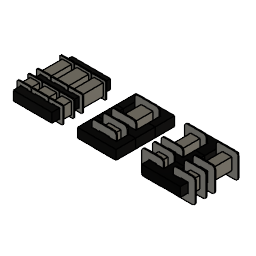
coil_formers (Autodesk Fusion 360 design; units mm, degrees)
Autodesk Fusion 360 part; units mm, degrees
sketch "Sketch1" plane through (0, 0, 0) normal (0, 0, 1) x (1, 0, 0) in component "Core"
  line L0 (0, 0) -> (30, 0)
  line L1 (30, 0) -> (30, 15.2)
  line L2 (30, 15.2) -> (0, 15.2)
  line L3 (0, 15.2) -> (0, 0)
  line L4 (15, 15.2) -> (15, 0) construction
  line L5 (11.4, 0) -> (5.25, 0)
  line L6 (5.25, 0) -> (5.25, 9.7)
  line L7 (5.25, 9.7) -> (11.4, 9.7)
  line L8 (11.4, 9.7) -> (11.4, 0)
  line L9 (24.75, 0) -> (24.75, 9.7)
  line L10 (24.75, 9.7) -> (18.6, 9.7)
  line L11 (18.6, 9.7) -> (18.6, 0)
  dimension "d7" = 30
  dimension "d8" = 15.2
  dimension "d9" = 9.7
  dimension "d10" = 7.2
  dimension "d11" = 19.5
  dimension "d36" = 5.25
  constraint horizontal L0
  constraint vertical L1
  constraint horizontal L2
  constraint vertical L3
  constraint coincident L0.start L3.end
  constraint midpoint L2 L4.start
  constraint midpoint L0 L4.end
  constraint horizontal L5
  constraint vertical L6
  constraint horizontal L7
  constraint vertical L8
  constraint coincident L0 L5.start
  constraint symmetric L4 L5.start L11.end
  constraint symmetric L4 L5.end L9.start
  constraint symmetric L4 L6.end L9.end
  constraint symmetric L4 L7.end L10.end
  measures "d7" distance of L0.start L0.end
  measures "d8" distance of L0.start L2.end
  measures "d9" distance of L5.end L6.end
  measures "d10" distance of L8 L11
  measures "d11" distance of L6 L9
  measures "d36" distance of L3 L6
extrude "Extrude1" add sketch "Sketch1" along normal blind 7.3 contours L0 L1 L2 L3 L6 L7 L8 L9 L10 L11 makes body 1 in component "Core"
sketch "Sketch1 (2)" plane through (0, 0, 0) normal (0, 1, 0) x (1, 0, 0) in component "Former_Center_Full"
  line L0 (3.85, 3.9) -> (-3.85, 3.9)
  line L1 (-3.85, 3.9) -> (-3.85, -3.9)
  line L2 (-3.85, -3.9) -> (3.85, -3.9)
  line L3 (3.85, -3.9) -> (3.85, 3.9)
  line L4 (3.85, 3.9) -> (-3.85, -3.9) construction
  line L5 (-3.85, 3.9) -> (3.85, -3.9) construction
  line L6 (-4.6, 4.65) -> (-4.6, -4.65)
  line L7 (-4.6, -4.65) -> (4.6, -4.65)
  line L8 (4.6, -4.65) -> (4.6, 4.65)
  line L9 (4.6, 4.65) -> (-4.6, 4.65)
  line L10 (6.55, 6.6) -> (-6.55, 6.6)
  line L11 (-6.55, 6.6) -> (-6.55, -6.6)
  line L12 (-6.55, -6.6) -> (6.55, -6.6)
  line L13 (6.55, -6.6) -> (6.55, 6.6)
  line L14 (6.55, 6.6) -> (-6.55, -6.6) construction
  line L15 (-6.55, 6.6) -> (6.55, -6.6) construction
  dimension "d19" = 7.8
  dimension "d20" = 7.7
  dimension "d21" = 0.75
  dimension "d22" = 13.1
  dimension "d24" = 1.95
  dimension "d25" = 1.95
  constraint horizontal L0
  constraint perpendicular L0 L1
  constraint parallel L0 L2
  constraint parallel L1 L3
  constraint coincident L4 origin
  constraint coincident L5 origin
  constraint horizontal L10
  constraint perpendicular L10 L11
  constraint parallel L10 L12
  constraint parallel L11 L13
  constraint coincident L14 origin
  constraint coincident L15 origin
  measures "d19" distance of L0.end L1.end
  measures "d20" distance of L1.end L2.end
  measures "d22" distance of L11.end L12.end
  measures "d24" distance of L8 L13
  measures "d25" distance of L9 L10
extrude "Extrude1'" add sketch "Sketch1 (2)" along normal blind 9.45 separate body contours L6 L7 L8 L9 makes body 2 in component "Former_Center_Full"
extrude "Extrude2" add sketch "Sketch1 (2)" along normal blind 0.75 contours L10 L11 L12 L13 bodies 2 in component "Former_Center_Full"
mirror "Mirror1" about plane through (0, 9.45, 0) normal (0, 1, 0) of bodies 2 merged in component "Former_Center_Full"
sketch "Sketch1 (3)" plane through (0, 0, 0) normal (0, 1, 0) x (1, 0, 0) in component "Former_Outer_Full"
  line L0 (2.875, 3.9) -> (-2.875, 3.9)
  line L1 (-2.875, 3.9) -> (-2.875, -3.9)
  line L2 (-2.875, -3.9) -> (2.875, -3.9)
  line L3 (2.875, -3.9) -> (2.875, 3.9)
  line L4 (2.875, 3.9) -> (-2.875, -3.9) construction
  line L5 (-2.875, 3.9) -> (2.875, -3.9) construction
  line L6 (-3.625, 4.65) -> (-3.625, -4.65)
  line L7 (-3.625, -4.65) -> (3.625, -4.65)
  line L8 (3.625, -4.65) -> (3.625, 4.65)
  line L9 (3.625, 4.65) -> (-3.625, 4.65)
  line L10 (5.575, 6.6) -> (-5.575, 6.6)
  line L11 (-5.575, 6.6) -> (-5.575, -6.6)
  line L12 (-5.575, -6.6) -> (5.575, -6.6)
  line L13 (5.575, -6.6) -> (5.575, 6.6)
  line L14 (5.575, 6.6) -> (-5.575, -6.6) construction
  line L15 (-5.575, 6.6) -> (5.575, -6.6) construction
  dimension "d19_1" = 7.8
  dimension "d20_1" = 5.75
  dimension "d21_1" = 0.75
  dimension "d24_1" = 1.95
  dimension "d25_1" = 1.95
  dimension "d37" = 1.95
  constraint horizontal L0
  constraint perpendicular L0 L1
  constraint parallel L0 L2
  constraint parallel L1 L3
  constraint coincident L4 origin
  constraint coincident L5 origin
  constraint horizontal L10
  constraint perpendicular L10 L11
  constraint parallel L10 L12
  constraint parallel L11 L13
  constraint coincident L14 origin
  constraint coincident L15 origin
  measures "d19_1" distance of L0.end L1.end
  measures "d20_1" distance of L1.end L2.end
  measures "d24_1" distance of L8 L13
  measures "d25_1" distance of L9 L10
  measures "d37" distance of L8 L13
extrude "Extrude1''" add sketch "Sketch1 (3)" along normal blind 9.45 separate body contours L6 L7 L8 L9 makes body 3 in component "Former_Outer_Full"
extrude "Extrude2'" add sketch "Sketch1 (3)" along normal blind 0.75 contours L10 L11 L12 L13 bodies 3 in component "Former_Outer_Full"
mirror "Mirror1'" about plane through (0, 9.45, 0) normal (0, 1, 0) of bodies 3 merged in component "Former_Outer_Full"
sketch "Sketch1 (4)" plane through (0, 0, 0) normal (0, 1, 0) x (1, 0, 0) in component "Former_Center_Half"
  line L0 (3.85, 3.9) -> (-3.85, 3.9)
  line L1 (-3.85, 3.9) -> (-3.85, -3.9)
  line L2 (-3.85, -3.9) -> (3.85, -3.9)
  line L3 (3.85, -3.9) -> (3.85, 3.9)
  line L4 (3.85, 3.9) -> (-3.85, -3.9) construction
  line L5 (-3.85, 3.9) -> (3.85, -3.9) construction
  line L6 (-4.6, 4.65) -> (-4.6, -4.65)
  line L7 (-4.6, -4.65) -> (4.6, -4.65)
  line L8 (4.6, -4.65) -> (4.6, 4.65)
  line L9 (4.6, 4.65) -> (-4.6, 4.65)
  line L10 (6.55, 6.6) -> (-6.55, 6.6)
  line L11 (-6.55, 6.6) -> (-6.55, -6.6)
  line L12 (-6.55, -6.6) -> (6.55, -6.6)
  line L13 (6.55, -6.6) -> (6.55, 6.6)
  line L14 (6.55, 6.6) -> (-6.55, -6.6) construction
  line L15 (-6.55, 6.6) -> (6.55, -6.6) construction
  dimension "d19_2" = 7.8
  dimension "d20_2" = 7.7
  dimension "d21_2" = 0.75
  dimension "d22_1" = 13.1
  dimension "d24_2" = 1.95
  dimension "d25_2" = 1.95
  constraint horizontal L0
  constraint perpendicular L0 L1
  constraint parallel L0 L2
  constraint parallel L1 L3
  constraint coincident L4 origin
  constraint coincident L5 origin
  constraint horizontal L10
  constraint perpendicular L10 L11
  constraint parallel L10 L12
  constraint parallel L11 L13
  constraint coincident L14 origin
  constraint coincident L15 origin
  measures "d19_2" distance of L0.end L1.end
  measures "d20_2" distance of L1.end L2.end
  measures "d22_1" distance of L11.end L12.end
  measures "d24_2" distance of L8 L13
  measures "d25_2" distance of L9 L10
extrude "Extrude1'''" add sketch "Sketch1 (4)" along normal blind 4.6 separate body contours L6 L7 L8 L9 makes body 4 in component "Former_Center_Half"
extrude "Extrude2''" add sketch "Sketch1 (4)" along normal blind 0.75 contours L10 L11 L12 L13 bodies 4 in component "Former_Center_Half"
mirror "Mirror1''" about plane through (0, 4.6, 0) normal (0, 1, 0) of bodies 4 merged in component "Former_Center_Half"
sketch "Sketch1 (5)" plane through (0, 0, 0) normal (0, 1, 0) x (1, 0, 0) in component "Former_Outer_Half"
  line L0 (2.875, 3.9) -> (-2.875, 3.9)
  line L1 (-2.875, 3.9) -> (-2.875, -3.9)
  line L2 (-2.875, -3.9) -> (2.875, -3.9)
  line L3 (2.875, -3.9) -> (2.875, 3.9)
  line L4 (2.875, 3.9) -> (-2.875, -3.9) construction
  line L5 (-2.875, 3.9) -> (2.875, -3.9) construction
  line L6 (-3.625, 4.65) -> (-3.625, -4.65)
  line L7 (-3.625, -4.65) -> (3.625, -4.65)
  line L8 (3.625, -4.65) -> (3.625, 4.65)
  line L9 (3.625, 4.65) -> (-3.625, 4.65)
  line L10 (5.575, 6.6) -> (-5.575, 6.6)
  line L11 (-5.575, 6.6) -> (-5.575, -6.6)
  line L12 (-5.575, -6.6) -> (5.575, -6.6)
  line L13 (5.575, -6.6) -> (5.575, 6.6)
  line L14 (5.575, 6.6) -> (-5.575, -6.6) construction
  line L15 (-5.575, 6.6) -> (5.575, -6.6) construction
  dimension "d19_1_1" = 7.8
  dimension "d20_1_1" = 5.75
  dimension "d21_1_1" = 0.75
  dimension "d24_1_1" = 1.95
  dimension "d25_1_1" = 1.95
  dimension "d37_1" = 1.95
  constraint horizontal L0
  constraint perpendicular L0 L1
  constraint parallel L0 L2
  constraint parallel L1 L3
  constraint coincident L4 origin
  constraint coincident L5 origin
  constraint horizontal L10
  constraint perpendicular L10 L11
  constraint parallel L10 L12
  constraint parallel L11 L13
  constraint coincident L14 origin
  constraint coincident L15 origin
  measures "d19_1_1" distance of L0.end L1.end
  measures "d20_1_1" distance of L1.end L2.end
  measures "d24_1_1" distance of L8 L13
  measures "d25_1_1" distance of L9 L10
  measures "d37_1" distance of L8 L13
extrude "Extrude1''''" add sketch "Sketch1 (5)" along normal blind 4.6 separate body contours L6 L7 L8 L9 makes body 5 in component "Former_Outer_Half"
extrude "Extrude2'''" add sketch "Sketch1 (5)" along normal blind 0.75 contours L10 L11 L12 L13 bodies 5 in component "Former_Outer_Half"
mirror "Mirror1'''" about plane through (0, 4.6, 0) normal (0, 1, 0) of bodies 5 merged in component "Former_Outer_Half"
sketch "Sketch1 (6)" plane through (0, 0, 0) normal (0, 1, 0) x (1, 0, 0) in component "Former_Center_Full_Aw"
  line L0 (3.85, 3.9) -> (-3.85, 3.9)
  line L1 (-3.85, 3.9) -> (-3.85, -3.9)
  line L2 (-3.85, -3.9) -> (3.85, -3.9)
  line L3 (3.85, -3.9) -> (3.85, 3.9)
  line L4 (3.85, 3.9) -> (-3.85, -3.9) construction
  line L5 (-3.85, 3.9) -> (3.85, -3.9) construction
  line L6 (-4.6, 4.65) -> (-4.6, -4.65)
  line L7 (-4.6, -4.65) -> (4.6, -4.65)
  line L8 (4.6, -4.65) -> (4.6, 4.65)
  line L9 (4.6, 4.65) -> (-4.6, 4.65)
  line L10 (9.5, 9.55) -> (-9.5, 9.55)
  line L11 (-9.5, 9.55) -> (-9.5, -9.55)
  line L12 (-9.5, -9.55) -> (9.5, -9.55)
  line L13 (9.5, -9.55) -> (9.5, 9.55)
  line L14 (9.5, 9.55) -> (-9.5, -9.55) construction
  line L15 (-9.5, 9.55) -> (9.5, -9.55) construction
  dimension "d19_3" = 7.8
  dimension "d20_3" = 7.7
  dimension "d21_3" = 0.75
  dimension "d22_2" = 19
  dimension "d24_3" = 4.9
  dimension "d25_3" = 4.9
  constraint horizontal L0
  constraint perpendicular L0 L1
  constraint parallel L0 L2
  constraint parallel L1 L3
  constraint coincident L4 origin
  constraint coincident L5 origin
  constraint horizontal L10
  constraint perpendicular L10 L11
  constraint parallel L10 L12
  constraint parallel L11 L13
  constraint coincident L14 origin
  constraint coincident L15 origin
  measures "d19_3" distance of L0.end L1.end
  measures "d20_3" distance of L1.end L2.end
  measures "d22_2" distance of L11.end L12.end
  measures "d24_3" distance of L8 L13
  measures "d25_3" distance of L9 L10
extrude "Extrude1'''''" add sketch "Sketch1 (6)" along normal blind 9.45 separate body contours L6 L7 L8 L9 makes body 6 in component "Former_Center_Full_Aw"
extrude "Extrude2''''" add sketch "Sketch1 (6)" along normal blind 0.75 contours L10 L11 L12 L13 bodies 6 in component "Former_Center_Full_Aw"
mirror "Mirror1''''" about plane through (0, 9.45, 0) normal (0, 1, 0) of bodies 6 merged in component "Former_Center_Full_Aw"
sketch "Sketch1 (7)" plane through (0, 0, 0) normal (0, 1, 0) x (1, 0, 0) in component "Former_Center_Half_Aw"
  line L0 (3.85, 3.9) -> (-3.85, 3.9)
  line L1 (-3.85, 3.9) -> (-3.85, -3.9)
  line L2 (-3.85, -3.9) -> (3.85, -3.9)
  line L3 (3.85, -3.9) -> (3.85, 3.9)
  line L4 (3.85, 3.9) -> (-3.85, -3.9) construction
  line L5 (-3.85, 3.9) -> (3.85, -3.9) construction
  line L6 (-4.6, 4.65) -> (-4.6, -4.65)
  line L7 (-4.6, -4.65) -> (4.6, -4.65)
  line L8 (4.6, -4.65) -> (4.6, 4.65)
  line L9 (4.6, 4.65) -> (-4.6, 4.65)
  line L10 (9.5, 9.55) -> (-9.5, 9.55)
  line L11 (-9.5, 9.55) -> (-9.5, -9.55)
  line L12 (-9.5, -9.55) -> (9.5, -9.55)
  line L13 (9.5, -9.55) -> (9.5, 9.55)
  line L14 (9.5, 9.55) -> (-9.5, -9.55) construction
  line L15 (-9.5, 9.55) -> (9.5, -9.55) construction
  dimension "d19_2_1" = 7.8
  dimension "d20_2_1" = 7.7
  dimension "d21_2_1" = 0.75
  dimension "d22_1_1" = 19
  dimension "d24_2_1" = 4.9
  dimension "d25_2_1" = 4.9
  constraint horizontal L0
  constraint perpendicular L0 L1
  constraint parallel L0 L2
  constraint parallel L1 L3
  constraint coincident L4 origin
  constraint coincident L5 origin
  constraint horizontal L10
  constraint perpendicular L10 L11
  constraint parallel L10 L12
  constraint parallel L11 L13
  constraint coincident L14 origin
  constraint coincident L15 origin
  measures "d19_2_1" distance of L0.end L1.end
  measures "d20_2_1" distance of L1.end L2.end
  measures "d22_1_1" distance of L11.end L12.end
  measures "d24_2_1" distance of L8 L13
  measures "d25_2_1" distance of L9 L10
extrude "Extrude1''''''" add sketch "Sketch1 (7)" along normal blind 4.6 separate body contours L6 L7 L8 L9 makes body 7 in component "Former_Center_Half_Aw"
extrude "Extrude2'''''" add sketch "Sketch1 (7)" along normal blind 0.75 contours L10 L11 L12 L13 bodies 7 in component "Former_Center_Half_Aw"
mirror "Mirror1'''''" about plane through (0, 4.6, 0) normal (0, 1, 0) of bodies 7 merged in component "Former_Center_Half_Aw"
fillet "Fillet1" radius 0.975 8 edges at (6.55, 18.525, -6.6) (-6.55, 18.525, -6.6) (6.55, 0.375, -6.6) (-6.55, 0.375, -6.6) (-6.55, 0.375, 6.6) (6.55, 0.375, 6.6) (-6.55, 18.525, 6.6) (6.55, 18.525, 6.6) on bodies 2 in component "Former_Center_Full"
fillet "Fillet1'" radius 0.975 8 edges at (-5.575, 0.375, -6.6) (5.575, 0.375, -6.6) (5.575, 18.525, -6.6) (-5.575, 18.525, -6.6) (-5.575, 0.375, 6.6) (5.575, 0.375, 6.6) (5.575, 18.525, 6.6) (-5.575, 18.525, 6.6) on bodies 3 in component "Former_Outer_Full"
fillet "Fillet1''" radius 0.975 8 edges at (-6.55, 0.375, 6.6) (-6.55, 8.825, 6.6) (6.55, 8.825, 6.6) (6.55, 0.375, 6.6) (-6.55, 8.825, -6.6) (-6.55, 0.375, -6.6) (6.55, 0.375, -6.6) (6.55, 8.825, -6.6) on bodies 4 in component "Former_Center_Half"
fillet "Fillet1'''" radius 0.975 8 edges at (-5.575, 8.825, 6.6) (5.575, 8.825, 6.6) (5.575, 0.375, 6.6) (-5.575, 0.375, 6.6) (-5.575, 8.825, -6.6) (-5.575, 0.375, -6.6) (5.575, 0.375, -6.6) (5.575, 8.825, -6.6) on bodies 5 in component "Former_Outer_Half"
fillet "Fillet1''''" radius 2.45 8 edges at (-9.5, 18.525, 9.55) (9.5, 18.525, 9.55) (-9.5, 0.375, 9.55) (9.5, 0.375, 9.55) (-9.5, 18.525, -9.55) (-9.5, 0.375, -9.55) (9.5, 0.375, -9.55) (9.5, 18.525, -9.55) on bodies 6 in component "Former_Center_Full_Aw"
fillet "Fillet1'''''" radius 2.45 8 edges at (-9.5, 0.375, -9.55) (-9.5, 8.825, -9.55) (9.5, 8.825, -9.55) (9.5, 0.375, -9.55) (9.5, 8.825, 9.55) (-9.5, 8.825, 9.55) (-9.5, 0.375, 9.55) (9.5, 0.375, 9.55) on bodies 7 in component "Former_Center_Half_Aw"
sketch "Sketch1 (8)" plane through (0, 0, 0) normal (0, 1, 0) x (1, 0, 0) in component "Former_Outer_Half (1)"
  line L0 (2.875, 3.9) -> (-2.875, 3.9)
  line L1 (-2.875, 3.9) -> (-2.875, -3.9)
  line L2 (-2.875, -3.9) -> (2.875, -3.9)
  line L3 (2.875, -3.9) -> (2.875, 3.9)
  line L4 (2.875, 3.9) -> (-2.875, -3.9) construction
  line L5 (-2.875, 3.9) -> (2.875, -3.9) construction
  line L6 (-3.625, 4.65) -> (-3.625, -4.65)
  line L7 (-3.625, -4.65) -> (3.625, -4.65)
  line L8 (3.625, -4.65) -> (3.625, 4.65)
  line L9 (3.625, 4.65) -> (-3.625, 4.65)
  line L10 (8.525, 9.55) -> (-8.525, 9.55)
  line L11 (-8.525, 9.55) -> (-8.525, -9.55)
  line L12 (-8.525, -9.55) -> (8.525, -9.55)
  line L13 (8.525, -9.55) -> (8.525, 9.55)
  line L14 (8.525, 9.55) -> (-8.525, -9.55) construction
  line L15 (-8.525, 9.55) -> (8.525, -9.55) construction
  dimension "d19_1_1_1" = 7.8
  dimension "d20_1_1_1" = 5.75
  dimension "d21_1_1_1" = 0.75
  dimension "d24_1_1_1" = 4.9
  dimension "d25_1_1_1" = 4.9
  dimension "d37_1_1" = 4.9
  constraint horizontal L0
  constraint perpendicular L0 L1
  constraint parallel L0 L2
  constraint parallel L1 L3
  constraint coincident L4 origin
  constraint coincident L5 origin
  constraint horizontal L10
  constraint perpendicular L10 L11
  constraint parallel L10 L12
  constraint parallel L11 L13
  constraint coincident L14 origin
  constraint coincident L15 origin
  measures "d19_1_1_1" distance of L0.end L1.end
  measures "d20_1_1_1" distance of L1.end L2.end
  measures "d24_1_1_1" distance of L8 L13
  measures "d25_1_1_1" distance of L9 L10
  measures "d37_1_1" distance of L8 L13
extrude "Extrude1'''''''" add sketch "Sketch1 (8)" along normal blind 4.6 separate body contours L6 L7 L8 L9 makes body 8 in component "Former_Outer_Half (1)"
extrude "Extrude2''''''" add sketch "Sketch1 (8)" along normal blind 0.75 contours L10 L11 L12 L13 bodies 8 in component "Former_Outer_Half (1)"
mirror "Mirror1''''''" about plane through (0, 4.6, 0) normal (0, 1, 0) of bodies 8 merged in component "Former_Outer_Half (1)"
fillet "Fillet1''''''" radius 2.45 8 edges at (-8.525, 8.825, 9.55) (8.525, 8.825, 9.55) (8.525, 0.375, 9.55) (-8.525, 0.375, 9.55) (-8.525, 8.825, -9.55) (-8.525, 0.375, -9.55) (8.525, 0.375, -9.55) (8.525, 8.825, -9.55) on bodies 8 in component "Former_Outer_Half (1)"
sketch "Sketch1 (9)" plane through (0, 0, 0) normal (0, 1, 0) x (1, 0, 0) in component "Former_Outer_Full (1)"
  line L0 (2.875, 3.9) -> (-2.875, 3.9)
  line L1 (-2.875, 3.9) -> (-2.875, -3.9)
  line L2 (-2.875, -3.9) -> (2.875, -3.9)
  line L3 (2.875, -3.9) -> (2.875, 3.9)
  line L4 (2.875, 3.9) -> (-2.875, -3.9) construction
  line L5 (-2.875, 3.9) -> (2.875, -3.9) construction
  line L6 (-3.625, 4.65) -> (-3.625, -4.65)
  line L7 (-3.625, -4.65) -> (3.625, -4.65)
  line L8 (3.625, -4.65) -> (3.625, 4.65)
  line L9 (3.625, 4.65) -> (-3.625, 4.65)
  line L10 (8.525, 9.55) -> (-8.525, 9.55)
  line L11 (-8.525, 9.55) -> (-8.525, -9.55)
  line L12 (-8.525, -9.55) -> (8.525, -9.55)
  line L13 (8.525, -9.55) -> (8.525, 9.55)
  line L14 (8.525, 9.55) -> (-8.525, -9.55) construction
  line L15 (-8.525, 9.55) -> (8.525, -9.55) construction
  dimension "d19_1_2" = 7.8
  dimension "d20_1_2" = 5.75
  dimension "d21_1_2" = 0.75
  dimension "d24_1_2" = 4.9
  dimension "d25_1_2" = 4.9
  dimension "d37_2" = 4.9
  constraint horizontal L0
  constraint perpendicular L0 L1
  constraint parallel L0 L2
  constraint parallel L1 L3
  constraint coincident L4 origin
  constraint coincident L5 origin
  constraint horizontal L10
  constraint perpendicular L10 L11
  constraint parallel L10 L12
  constraint parallel L11 L13
  constraint coincident L14 origin
  constraint coincident L15 origin
  measures "d19_1_2" distance of L0.end L1.end
  measures "d20_1_2" distance of L1.end L2.end
  measures "d24_1_2" distance of L8 L13
  measures "d25_1_2" distance of L9 L10
  measures "d37_2" distance of L8 L13
extrude "Extrude1''''''''" add sketch "Sketch1 (9)" along normal blind 9.45 separate body contours L6 L7 L8 L9 makes body 9 in component "Former_Outer_Full (1)"
extrude "Extrude2'''''''" add sketch "Sketch1 (9)" along normal blind 0.75 contours L10 L11 L12 L13 bodies 9 in component "Former_Outer_Full (1)"
mirror "Mirror1'''''''" about plane through (0, 9.45, 0) normal (0, 1, 0) of bodies 9 merged in component "Former_Outer_Full (1)"
fillet "Fillet1'''''''" radius 2.45 8 edges at (-8.525, 0.375, -9.55) (8.525, 0.375, -9.55) (8.525, 18.525, -9.55) (-8.525, 18.525, -9.55) (-8.525, 0.375, 9.55) (8.525, 0.375, 9.55) (8.525, 18.525, 9.55) (-8.525, 18.525, 9.55) on bodies 9 in component "Former_Outer_Full (1)"
component "Core 1" placed x (1, 0, 0) y (0, 1, 0) z (0, 0, 1) at (0, 0, 0)
component "Core 2" placed x (1, 0, 0) y (0, 1, 0) z (0, 0, 1) at (0, 0, 0)
component "Core 3" placed x (1, 0, 0) y (0, 1, 0) z (0, 0, 1) at (0, 0, 0)
component "Core" placed x (1, 0, 0) y (0, -1, 0) z (0, 0, -1) at (0, 0, 7.3) in component "Core 1"
component "Core" placed x (1, 0, 0) y (0, -1, 0) z (0, 0, -1) at (0, -15.2, 7.3) in component "Core 1"
component "Core" placed x (1, 0, 0) y (0, 1, 0) z (0, 0, 1) at (0, 0, 0) in component "Core 1"
component "Former_Center_Full" placed x (1, 0, 0) y (0, 1, 0) z (0, 0, 1) at (15, -9.45, 3.65) in component "Core 1"
component "Former_Outer_Half" placed x (1, 0, 0) y (0, 1, 0) z (0, 0, 1) at (2.625, -24.65, 3.65) in component "Core 1"
component "Former_Center_Half" placed x (1, 0, 0) y (0, 1, 0) z (0, 0, 1) at (15, -24.65, 3.65) in component "Core 1"
component "Former_Outer_Full" placed x (1, 0, 0) y (0, 1, 0) z (0, 0, 1) at (2.625, -9.45, 3.65) in component "Core 1"
component "Former_Outer_Half" placed x (1, 0, 0) y (0, 1, 0) z (0, 0, 1) at (27.375, -24.65, 3.65) in component "Core 1"
component "Former_Outer_Full" placed x (1, 0, 0) y (0, 1, 0) z (0, 0, 1) at (27.375, -9.45, 3.65) in component "Core 1"
component "Core" placed x (1, 0, 0) y (0, -1, 0) z (0, 0, -1) at (50, -15.2, 7.3) in component "Core 2"
component "Core" placed x (1, 0, 0) y (0, -1, 0) z (0, 0, -1) at (50, 0, 7.3) in component "Core 2"
component "Core" placed x (1, 0, 0) y (0, 1, 0) z (0, 0, 1) at (50, 0, 0) in component "Core 2"
component "Former_Center_Full_Aw" placed x (1, 0, 0) y (0, 1, 0) z (0, 0, 1) at (65, -9.45, 3.65) in component "Core 2"
component "Former_Center_Half_Aw" placed x (1, 0, 0) y (0, 1, 0) z (0, 0, 1) at (65, -24.65, 3.65) in component "Core 2"
component "Core" placed x (1, 0, 0) y (0, 1, 0) z (0, 0, 1) at (100, 0, 0) in component "Core 3"
component "Core" placed x (1, 0, 0) y (0, -1, 0) z (0, 0, -1) at (100, 0, 7.3) in component "Core 3"
component "Former_Outer_Full (1)" placed x (1, 0, 0) y (0, 1, 0) z (0, 0, 1) at (102.625, -9.45, 3.65) in component "Core 3"
component "Former_Outer_Half (1)" placed x (1, 0, 0) y (0, 1, 0) z (0, 0, 1) at (102.625, -24.65, 3.65) in component "Core 3"
component "Core" placed x (1, 0, 0) y (0, -1, 0) z (0, 0, -1) at (100, -15.2, 7.3) in component "Core 3"
component "Former_Outer_Half (1)" placed x (1, 0, 0) y (0, 1, 0) z (0, 0, 1) at (127.375, -24.65, 3.65) in component "Core 3"
component "Former_Outer_Full (1)" placed x (1, 0, 0) y (0, 1, 0) z (0, 0, 1) at (127.375, -9.45, 3.65) in component "Core 3"
equation "Core_W = 30 mm"
equation "Core_L = 15.2 mm"
equation "Core_H = 7.3 mm"
equation "Core_Center_W = 7.2 mm"
equation "Core_Outer_Sep = 19.5 mm"
equation "Core_Window_L = 9.7 mm"
equation "d7 = Core_W"
equation "d8 = Core_L"
equation "d9 = Core_Window_L"
equation "d10 = Core_Center_W"
equation "d11 = Core_Outer_Sep"
equation "d12 = Core_H"
equation "Spacing = 0.25 mm"
equation "Thickness = 0.75 mm"
equation "d19 = Core_H + 2 * Spacing"
equation "d20 = Core_Center_W + 2 * Spacing"
equation "d21 = Thickness"
equation "d22 = ( Core_Outer_Sep - Core_Center_W ) / 2 + Core_Center_W - Spacing"
equation "d25 = d24"
equation "d26 = Core_Window_L - Spacing"
equation "d28 = Thickness"
equation "d33 = -Spacing"
equation "d34 = Spacing"
equation "d35 = Spacing"
equation "d19_1 = Core_H + 2 * Spacing"
equation "d20_1 = d36 + 2 * Spacing"
equation "d21_1 = Thickness"
equation "d25_1 = d24_1"
equation "d26_1 = Core_Window_L - Spacing"
equation "d28_1 = Thickness"
equation "d37 = d24"
equation "d39 = Spacing"
equation "d40 = -Spacing"
equation "d41 = -Spacing"
equation "d19_2 = Core_H + 2 * Spacing"
equation "d20_2 = Core_Center_W + 2 * Spacing"
equation "d21_2 = Thickness"
equation "d22_1 = ( Core_Outer_Sep - Core_Center_W ) / 2 + Core_Center_W - Spacing"
equation "d25_2 = d24_2"
equation "d26_2 = Core_Window_L / 2 - Spacing"
equation "d28_2 = Thickness"
equation "d19_1_1 = Core_H + 2 * Spacing"
equation "d20_1_1 = d36 + 2 * Spacing"
equation "d21_1_1 = Thickness"
equation "d25_1_1 = d24_1_1"
equation "d26_1_1 = Core_Window_L / 2 - Spacing"
equation "d28_1_1 = Thickness"
equation "d37_1 = d24"
equation "d51 = Spacing"
equation "d52 = -Spacing"
equation "d53 = Spacing"
equation "d55 = Spacing"
equation "d56 = Spacing"
equation "d57 = -Spacing"
equation "d19_3 = Core_H + 2 * Spacing"
equation "d20_3 = Core_Center_W + 2 * Spacing"
equation "d21_3 = Thickness"
equation "d22_2 = Core_Outer_Sep - 2 * Spacing"
equation "d25_3 = d24_3"
equation "d26_3 = Core_Window_L - Spacing"
equation "d28_3 = Thickness"
equation "d59 = Spacing"
equation "d60 = -Spacing"
equation "d61 = Spacing"
equation "d19_2_1 = Core_H + 2 * Spacing"
equation "d20_2_1 = Core_Center_W + 2 * Spacing"
equation "d21_2_1 = Thickness"
equation "d22_1_1 = Core_Outer_Sep - 2 * Spacing"
equation "d25_2_1 = d24_2_1"
equation "d26_2_1 = Core_Window_L / 2 - Spacing"
equation "d28_2_1 = Thickness"
equation "d63 = Spacing"
equation "d64 = -Spacing"
equation "d65 = Spacing"
equation "d67 = d24 / 2"
equation "d69 = d24_1 / 2"
equation "d71 = d24_2 / 2"
equation "d73 = d24_1_1 / 2"
equation "d75 = d24_3 / 2"
equation "d77 = d24_2_1 / 2"
equation "d19_1_1_1 = Core_H + 2 * Spacing"
equation "d20_1_1_1 = d36 + 2 * Spacing"
equation "d21_1_1_1 = Thickness"
equation "d25_1_1_1 = d24_1_1_1"
equation "d26_1_1_1 = Core_Window_L / 2 - Spacing"
equation "d28_1_1_1 = Thickness"
equation "d37_1_1 = d24_3"
equation "d73_1 = d24_1_1_1 / 2"
equation "d19_1_2 = Core_H + 2 * Spacing"
equation "d20_1_2 = d36 + 2 * Spacing"
equation "d21_1_2 = Thickness"
equation "d25_1_2 = d24_1_2"
equation "d26_1_2 = Core_Window_L - Spacing"
equation "d28_1_2 = Thickness"
equation "d37_2 = d24_3"
equation "d69_1 = d24_1_2 / 2"
equation "d111 = Spacing"
equation "d112 = -Spacing"
equation "d113 = -Spacing"
equation "d115 = Spacing"
equation "d116 = -Spacing"
equation "d117 = -Spacing"
equation "d119 = Spacing"
equation "d120 = -Spacing"
equation "d121 = Spacing"
equation "d123 = Spacing"
equation "d124 = -Spacing"
equation "d125 = Spacing"
equation "d127 = Spacing"
equation "d128 = -Spacing"
equation "d129 = Spacing"
equation "d131 = Spacing"
equation "d132 = -Spacing"
equation "d133 = Spacing"
